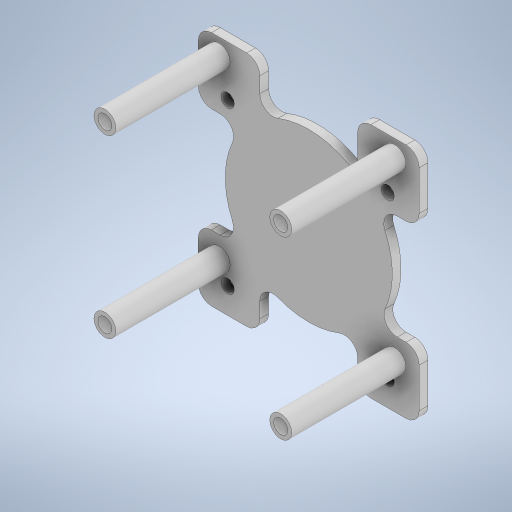
# Autodesk Inventor part: soporteHBridge
Saved by Autodesk Inventor 2023.1 (Build 271208000, 208)
## iProperties
Created: 2023-05-11
Part Number: soporteHBridge
Material: Generic
Document SubType Name: Modeling
Designer: felip
Density: 1 g/cm^3
Appearance: Default
Author: felip
Autodesk Inventor part; units mm, degrees
ref_plane "YZ Plane" through (0, 0, 0) normal (1, 0, 0) x (0, 1, 0)
ref_plane "XZ Plane" through (0, 0, 0) normal (0, 1, 0) x (-1, 0, 0)
ref_plane "Work Plane1" through (0, 0, 0) normal (0, 0, 1) x (1, 0, 0)
sketch "Sketch1" plane through (0, 0, 0) normal (0, 0, 1) x (1, 0, 0)
  circle A0 centre (22.2, -27.45) radius 1.5 projected
  circle A1 centre (58.6, -27.45) radius 1.5 projected
  circle A2 centre (22.2, 9.15) radius 1.5 projected
  circle A3 centre (58.6, 9.15) radius 1.5 projected
  line L0 (15.5, 16.5) -> (15.5, -25.3) projected
  line L1 (19.5, -29.3) -> (61, -29.3) projected
  line L2 (61, 20.5) -> (19.5, 20.5) projected
  line L3 (64.8607, 14) -> (64.8607, -18) projected
  line L4 (65.75, -18) -> (65.75, 14) projected
  line L5 (65.75, -33.3) -> (51.75, -33.3)
  line L6 (51.75, -33.3) -> (51.75, -21.8024)
  line L7 (55.4368, -18.3) -> (65.75, -18.3)
  line L8 (65.75, -18.3) -> (65.75, -33.3)
  line L9 (15.5, -33.3) -> (29.5, -33.3)
  line L10 (29.5, -33.3) -> (29.5, -21.8024)
  line L11 (25.8132, -18.3) -> (15.5, -18.3)
  line L12 (15.5, -18.3) -> (15.5, -33.3)
  line L13 (15.5, 20.5697) -> (29.5, 20.5697)
  line L14 (29.5, 20.5697) -> (29.5, 9.0024)
  line L15 (25.8695, 5.5697) -> (15.5, 5.5697)
  line L16 (15.5, 5.5697) -> (15.5, 20.5697)
  line L17 (51.75, 20.5697) -> (65.75, 20.5697)
  line L18 (65.75, 20.5697) -> (65.75, 5.5697)
  line L19 (65.75, 5.5697) -> (55.3805, 5.5697)
  line L20 (51.75, 9.0024) -> (51.75, 20.5697)
  arc A4 (51.75, 9.0024) -> (29.5, 9.0024) centre (40.625, -6.4) ccw
  arc A5 (25.8695, 5.5697) -> (25.8132, -18.3) centre (40.625, -6.4) ccw
  arc A6 (29.5, -21.8024) -> (51.75, -21.8024) centre (40.625, -6.4) ccw
  arc A7 (55.4368, -18.3) -> (55.3805, 5.5697) centre (40.625, -6.4) ccw
  line L21 (65.75, 20.5697) -> (65.75, 5.5697)
  line L22 (65.75, -18.3) -> (65.75, -33.3)
  line L23 (15.5, 20.5697) -> (29.5, 20.5697)
  line L24 (51.75, 20.5697) -> (65.75, 20.5697)
  line L25 (15.5, -33.3) -> (15.5, -18.3)
  line L26 (15.5, 5.5697) -> (15.5, 20.5697)
  point P0 (0, 0)
  point P1 (40.25, 20.5)
  dimension "d10" = 50.25
  dimension "d13" = 26.9
  constraints: 44 end point, 12 parallel, 8 perpendicular, 8 point on circle, 6 horizontal, 4 centre point, 1 midpoint, 1 point on line
  measures "d10" distance of L5.start L9.start
  measures "d13" distance from line of L2 A4.centre
extrude "Extrusion1" add sketch "Sketch1" along normal blind 2 contours L16 L13 L14 A4 L20 L17 L18 L4 L19 A7 L7 L8 L5 L6 A6 L10 L9 L12 L0 L11 A5 L15
fillet "Fillet1" radius 3 7 edges at (55.3805, 5.5697, 1) (29.5, -21.8024, 1) (25.8132, -18.3, 1) (29.5, 9.0024, 1) (55.4368, -18.3, 1) (25.8695, 5.5697, 1) (51.75, -21.8024, 1)
fillet "Fillet2" radius 3 12 edges at (15.5, 20.5697, 1) (15.5, 5.5697, 1) (29.5, 20.5697, 1) (51.75, 20.5697, 1) (65.75, 20.5697, 1) (65.75, -18.3, 1) (51.75, -33.3, 1) (15.5, -18.3, 1) (15.5, -33.3, 1) (29.5, -33.3, 1) (65.75, -33.3, 1) (65.75, 5.5697, 1)
sketch "Sketch2" plane through (0, 0, 2) normal (0, 0, 1) x (1, 0, 0)
  circle A0 centre (60.25, -23.1) radius 1.6 projected
  circle A1 centre (20.25, -23.1) radius 1.6 projected
  circle A2 centre (20.25, 16.9) radius 1.6 projected
  circle A3 centre (60.25, 16.9) radius 1.6 projected
  circle A4 centre (20.25, -23.1) radius 2.5
  circle A5 centre (60.25, 16.9) radius 2.5
  circle A6 centre (20.25, 16.9) radius 2.5
  circle A7 centre (60.25, -23.1) radius 2.5
  point P0 (0, 0)
  dimension "d17" = 5
  dimension "d18" = 5
  dimension "d19" = 5
  dimension "d20" = 5
  constraints: 4 centre point, 4 coincident
  measures "d17" diameter of A4
  measures "d18" diameter of A5
  measures "d19" diameter of A6
  measures "d20" diameter of A7
extrude "Extrusion2" add sketch "Sketch2" along normal blind 26
equation "\"d13\" = 0.5 * d11"
equation "\"d11\" = 53.8"
body "Solid1"
